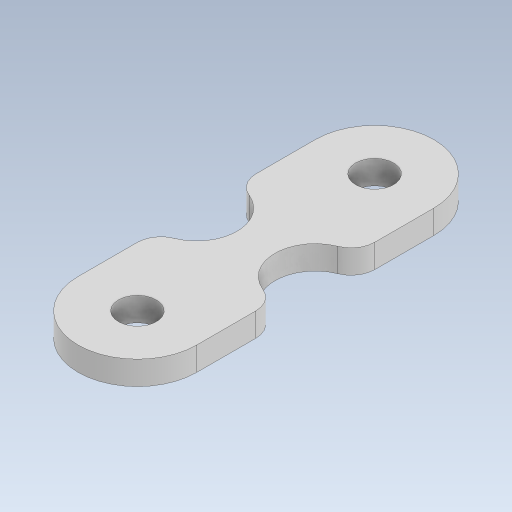
# Autodesk Inventor part: Fix Konektor Casis Kecil
Saved by Autodesk Inventor 2023.5 (Build 275446000, 446)
## iProperties
Created: 2025-10-17
Part Number: Fix Konektor Casis Kecil
Material: Generic
Document SubType Name: Modeling
Designer: Guntur
Density: 1 g/cm^3
Appearance: Default
Author: Guntur
Autodesk Inventor part; units mm, degrees
ref_plane "YZ Plane" through (0, 0, 0) normal (1, 0, 0) x (0, 1, 0)
ref_plane "XZ Plane" through (0, 0, 0) normal (0, 1, 0) x (-1, 0, 0)
ref_plane "XY Plane" through (0, 0, 0) normal (0, 0, 1) x (1, 0, 0)
sketch "Sketch1" plane through (0, 0, 0) normal (0, 1, 0) x (-1, 0, 0)
  circle A0 centre (0, 0) radius 1.6
  circle A1 centre (0, -20) radius 1.6
  line L0 (0, 0) -> (0, -20) construction
  arc A2 (5, 0) -> (-5, 0) centre (0, 0) ccw
  arc A3 (-5, -20) -> (5, -20) centre (0, -20) ccw
  arc A4 (-5, -13.4) -> (-5, -6.6) centre (-5, -10) ccw
  arc A5 (5, -6.6) -> (5, -13.4) centre (5, -10) ccw
  line L1 (5, -20) -> (5, -13.4)
  line L2 (5, -6.6) -> (5, 0)
  line L3 (-5, 0) -> (-5, -6.6)
  line L4 (-5, -13.4) -> (-5, -20)
  point P0 (0, -10)
  dimension "d0" = 3.2
  dimension "d1" = 3.2
  dimension "d2" = 20
  constraints: 12 end point, 8 point on circle, 8 tangent, 6 centre point, 4 parallel, 1 coincident, 1 midpoint, 1 vertical
  measures "d0" diameter of A0
  measures "d1" diameter of A1
  measures "d2" distance of L0.end point (0, 0)
extrude "Extrusion1" add sketch "Sketch1" along normal blind 2
fillet "Fillet1" radius 2 4 edges at (5, 1, -6.6) (5, 1, -13.4) (-5, 1, -6.6) (-5, 1, -13.4)
body "Solid1"
